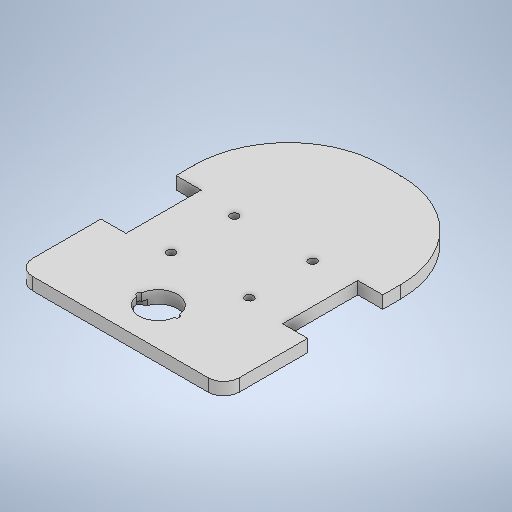
# Autodesk Inventor part: micromouse
Saved by Autodesk Inventor 2025 (Build 290162000, 162)
## iProperties
Created: 2026-04-22
Part Number: micromouse
Material: Generic
Document SubType Name: Modeling
Designer: dalto
Density: 1 g/cm^3
Appearance: Default
Author: dalto
Autodesk Inventor part; units mm, degrees
ref_plane "YZ Plane" through (0, 0, 0) normal (1, 0, 0) x (0, 1, 0)
ref_plane "XZ Plane" through (0, 0, 0) normal (0, 1, 0) x (-1, 0, 0)
ref_plane "XY Plane" through (0, 0, 0) normal (0, 0, 1) x (1, 0, 0)
sketch "Sketch1" plane through (0, 0, 0) normal (0, 1, 0) x (-1, 0, 0)
  line L0 (-35.56, 55) -> (35.56, 55)
  line L1 (41.91, 48.65) -> (41.91, -16.9)
  line L2 (3.81, -55) -> (-3.81, -55)
  line L3 (-41.91, -16.9) -> (-41.91, 48.65)
  line L4 (-41.91, 55) -> (41.91, -55) construction
  line L5 (41.91, 55) -> (-41.91, -55) construction
  arc A0 (3.81, -55) -> (41.91, -16.9) centre (3.81, -16.9) ccw
  arc A1 (-41.91, -16.9) -> (-3.81, -55) centre (-3.81, -16.9) ccw
  arc A2 (41.91, 48.65) -> (35.56, 55) centre (35.56, 48.65) ccw
  arc A3 (-35.56, 55) -> (-41.91, 48.65) centre (-35.56, 48.65) ccw
  line L6 (113.65, -53.500747) -> (-33.65, 85.250747) construction
  line L7 (-33.65, -53.500747) -> (113.65, 85.250747) construction
  line L8 (52.07, -9.508324) -> (31.75, -9.508324)
  line L9 (31.75, -9.508324) -> (31.75, 20.971676)
  line L10 (31.75, 20.971676) -> (52.07, 20.971676)
  line L11 (52.07, 20.971676) -> (52.07, -9.508324)
  line L12 (52.07, -9.508324) -> (31.75, 20.971676) construction
  line L13 (31.75, -9.508324) -> (52.07, 20.971676) construction
  line L14 (0, -55) -> (0, 55)
  line L15 (33.65, -53.500747) -> (-113.65, 85.250747) construction
  line L16 (-52.07, -9.508324) -> (-31.75, -9.508324)
  line L17 (-31.75, -9.508324) -> (-31.75, 20.971676)
  line L18 (-31.75, 20.971676) -> (-52.07, 20.971676)
  line L19 (-52.07, 20.971676) -> (-52.07, -9.508324)
  line L20 (-52.07, -9.508324) -> (-31.75, 20.971676) construction
  line L21 (-31.75, -9.508324) -> (-52.07, 20.971676) construction
  line L22 (-52.07, 20.971676) -> (-31.75, 20.971676)
  line L23 (-31.75, 20.971676) -> (-31.75, -9.508324)
  line L24 (-31.75, -9.508324) -> (-52.07, -9.508324)
  line L25 (-52.07, -9.508324) -> (-52.07, 20.971676)
  line L26 (-52.07, 20.971676) -> (-31.75, -9.508324) construction
  line L27 (-31.75, 20.971676) -> (-52.07, -9.508324) construction
  point P0 (0, 0)
  point P1 (-35.56, 48.65)
  point P2 (41.91, 5.731676)
  point P3 (-41.91, 5.731676)
  point P4 (-41.91, 5.731676)
  point P5 (41.91, -9.508324)
  point P6 (41.91, 20.971676)
  point P7 (-41.91, 20.971676)
  point P8 (-41.91, -9.508324)
  dimension "d0" = 83.82
  dimension "d1" = 110
  dimension "d2" = 38.1
  dimension "d3" = 38.1
  dimension "d4" = 6.35
  dimension "d5" = 6.35
  dimension "d11" = 20.32
  dimension "d12" = 30.48
  constraints: 56 end point, 9 midpoint, 9 point on line, 8 point on circle, 8 tangent, 7 symmetric about line, 6 parallel, 4 centre point, 3 horizontal, 3 perpendicular
  measures "d0" distance of L4.end L5.end
  measures "d1" distance of L5.start L4.end
  measures "d2" radius of A0
  measures "d3" radius of A1
  measures "d4" radius of A2
  measures "d5" radius of A3
  measures "d11" distance of L9.end L10.end
  measures "d12" distance of L8.end L9.end
extrude "Extrusion1" add sketch "Sketch1" along normal blind 5.08 contours L0 L14 L2 A1 L3 L16 L17 L18 A3 | L0 A2 L1 L10 L9 L8 A0 L2 L14
sketch "Sketch2" plane through (0, 0, 0) normal (0, -1, 0) x (1, 0, 0)
  line L0 (-35.56, 55) -> (35.56, 55)
  line L1 (0, 55) -> (0, 47.38)
  line L2 (0, 47.38) -> (0, 31.886)
  circle A0 centre (0, 39.633) radius 7.747
  line L3 (7.747, 39.633) -> (9.017, 39.633)
  circle A1 centre (9.017, 39.633) radius 1.27
  line L4 (9.756904, 38.600798) -> (7.196844, 36.765693) construction
  spline S0 degree 1 poles (9.756904, 38.600798) (7.196844, 36.765693) knots 1 1 2 2
  line L5 (9.770215, 40.65553) -> (7.167589, 42.572673) construction
  spline S1 degree 1 poles (9.770215, 40.65553) (7.167589, 42.572673) knots 1 1 2 2
  line L6 (-7.747, 39.633) -> (-9.017, 39.633)
  circle A2 centre (-9.017, 39.633) radius 1.27
  line L7 (-9.756904, 38.600798) -> (-7.196844, 36.765693) construction
  spline S2 degree 1 poles (-9.756904, 38.600798) (-7.196844, 36.765693) knots 1 1 2 2
  line L8 (-9.770215, 40.65553) -> (-7.167589, 42.572673) construction
  spline S3 degree 1 poles (-9.770215, 40.65553) (-7.167589, 42.572673) knots 1 1 2 2
  circle A3 centre (-9.017, 39.633) radius 1.27
  line L9 (-9.770215, 40.65553) -> (-7.167589, 42.572673) construction
  spline S4 degree 1 poles (-9.770215, 40.65553) (-7.167589, 42.572673) knots 1 1 2 2
  line L10 (-9.756904, 38.600798) -> (-7.196844, 36.765693) construction
  spline S5 degree 1 poles (-9.756904, 38.600798) (-7.196844, 36.765693) knots 1 1 2 2
  line L11 (10.287, 39.633) -> (10.287, 32.454774)
  line L12 (-10.287, 39.633) -> (-10.287, 31.176127)
  circle A4 centre (7.747, 39.633) radius 1.016
  line L13 (-7.747, 39.633) -> (-9.017, 39.633)
  circle A5 centre (-9.017, 39.633) radius 1.27
  circle A6 centre (-7.747, 39.633) radius 1.016
  circle A7 centre (-7.747, 39.633) radius 1.016
  point P0 (0, 0)
  dimension "d16" = 7.62
  dimension "d17" = 15.494
  dimension "d19" = 1.27
  dimension "d27" = 2.032
  dimension "d28" = 20.574
  constraints: 14 end point, 13 point on circle, 9 symmetric about line, 9 tangent, 7 centre point, 7 coincident, 4 vertical, 2 collinear, 2 midpoint, 1 concentric, 1 horizontal, 1 horizontal alignment, 23 other
  measures "d16" distance of L1.start L1.end
  measures "d17" distance of L1.end L2.end
  measures "d19" distance of L3.start L3.end
  measures "d27" diameter of A4
  measures "d28" horizontal distance of L12.end L11.end
extrude "Extrusion2" cut sketch "Sketch2" against normal blind 5.08 contours A0 A4 L2 | L2 A0 A6 | A0 A4 | A6 A0
sketch "Sketch7" plane through (0, 0, 0) normal (0, -1, 0) x (1, 0, 0)
  circle A0 centre (0, 39.633) radius 7.747
  line L0 (7.747, 39.633) -> (8.89, 39.633)
  circle A1 centre (8.89, 39.633) radius 1.143
  circle A2 centre (7.747, 39.633) radius 0.9525
  line L1 (9.653215, 40.483854) -> (7.169913, 42.566999) construction
  spline S0 degree 1 poles (9.653215, 40.483854) (7.169913, 42.566999) knots 1 1 2 2
  line L2 (9.653215, 38.782146) -> (7.169913, 36.699001) construction
  spline S1 degree 1 poles (9.653215, 38.782146) (7.169913, 36.699001) knots 1 1 2 2
  line L3 (0, 47.38) -> (0, 31.886)
  circle A3 centre (-8.89, 39.633) radius 1.143
  line L4 (-9.653215, 40.483854) -> (-7.169913, 42.566999) construction
  spline S2 degree 1 poles (-9.653215, 40.483854) (-7.169913, 42.566999) knots 1 1 2 2
  line L5 (-9.653215, 38.782146) -> (-7.169913, 36.699001) construction
  spline S3 degree 1 poles (-9.653215, 38.782146) (-7.169913, 36.699001) knots 1 1 2 2
  circle A4 centre (-8.89, 39.633) radius 1.143
  line L6 (-9.653215, 40.483854) -> (-7.169913, 42.566999) construction
  spline S4 degree 1 poles (-9.653215, 40.483854) (-7.169913, 42.566999) knots 1 1 2 2
  line L7 (-9.653215, 38.782146) -> (-7.169913, 36.699001) construction
  spline S5 degree 1 poles (-9.653215, 38.782146) (-7.169913, 36.699001) knots 1 1 2 2
  point P0 (0, 0)
  dimension "d40" = 1.143
  dimension "d41" = 1.905
  constraints: 10 point on circle, 5 symmetric about line, 4 centre point, 4 end point, 3 coincident, 2 collinear, 1 horizontal, 1 vertical, 19 other
  measures "d40" distance of L0.start L0.end
  measures "d41" diameter of A2
sketch "Sketch7 outline for Extrusion4" plane through (0, 0, 0) normal (0, -1, 0) x (1, 0, 0)
  spline S0 degree 1 poles (-9.653215, 40.483854) (-7.169913, 42.566999) knots 0 0 1 1
  arc A0 (-7.169913, 36.699001) -> (-7.169913, 42.566999) centre (0, 39.633) cw
  spline S1 degree 1 poles (-9.653215, 38.782146) (-7.169913, 36.699001) knots 0 0 1 1
  arc A1 (-9.653215, 40.483854) -> (-9.653215, 38.782146) centre (-8.89, 39.633) ccw
  spline S2 degree 1 poles (9.653215, 40.483854) (7.169913, 42.566999) knots 0 0 1 1
  arc A2 (9.653215, 38.782146) -> (9.653215, 40.483854) centre (8.89, 39.633) ccw
  spline S3 degree 1 poles (9.653215, 38.782146) (7.169913, 36.699001) knots 0 0 1 1
  arc A3 (7.169913, 42.566999) -> (7.169913, 36.699001) centre (0, 39.633) cw
extrude "Extrusion4" cut sketch "Sketch7 outline for Extrusion4" against normal blind 2.032
sketch "Sketch8" plane through (0, 0, 0) normal (0, -1, 0) x (1, 0, 0)
  arc A0 (7.169913, 36.699001) -> (7.169913, 42.566999) centre (0, 39.633) ccw
  circle A1 centre (7.747, 39.633) radius 0.9525
  line L0 (0, 47.38) -> (0, 31.886)
  circle A2 centre (-7.747, 39.633) radius 0.9525
  circle A3 centre (-7.747, 39.633) radius 0.9525
  point P0 (0, 0)
  dimension "d44" = 1.905
  constraints: 3 centre point, 2 end point, 1 coincident, 1 concentric, 1 point on circle, 1 symmetric about line, 1 vertical, 1 other
  measures "d44" diameter of A1
extrude "Extrusion5" cut sketch "Sketch8" against normal blind 5.08
sketch "Sketch9" plane through (0, 0, 0) normal (0, -1, 0) x (1, 0, 0)
  line L0 (31.75, 20.971676) -> (31.75, -9.508324)
  line L1 (31.75, 5.731676) -> (10.338001, 5.731676)
  line L2 (0, 23.8125) -> (0, -11.1125)
  line L3 (15.875, 5.731676) -> (15.875, 18.558676)
  line L4 (41.91, 18.558676) -> (15.875, 18.558676)
  line L5 (41.91, 48.65) -> (41.91, 20.971676)
  circle A0 centre (15.875, 18.558676) radius 1.651
  circle A1 centre (15.875, -7.095324) radius 1.651
  circle A2 centre (-15.875, 18.558676) radius 1.651
  circle A3 centre (-15.875, -7.095324) radius 1.651
  point P0 (0, 0)
  dimension "d51" = 12.827
  dimension "d52" = 26.035
  dimension "d53" = 3.302
  constraints: 8 end point, 4 centre point, 3 symmetric about line, 1 coincident, 1 horizontal, 1 midpoint, 1 perpendicular, 1 point on line, 1 vertical, 3 other
  measures "d51" distance of L3.start L3.end
  measures "d52" distance of L4.start L3.end
  measures "d53" diameter of A0
extrude "Extrusion6" cut sketch "Sketch9" against normal blind 5.08 contours A0 L3 L4 | L4 L3 A0 | A1 | A2 | A3
body "Solid1"
